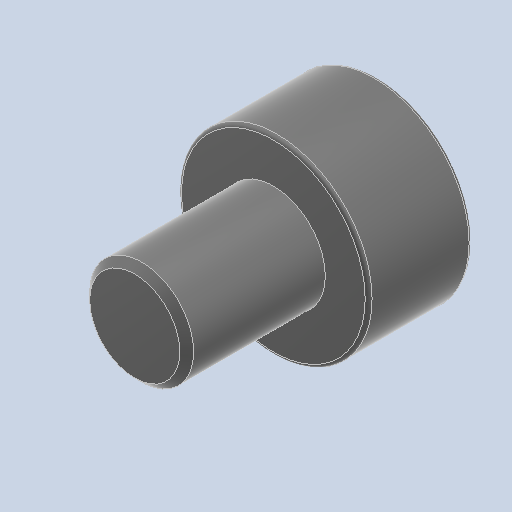
# Autodesk Inventor part: M3 x 4mm FHCS
Saved by Autodesk Inventor 2022 (Build 260153000, 153)
## iProperties
Created: 2021-10-06
Part Number: M3 x 4mm FHCS
Material: Stainless Steel
Document SubType Name: Modeling
Designer: Administrator
Density: 8 g/cm^3
Appearance: Smooth - Black
Mass: 0.890655 g
Surface Area: 1.98084 cm^2
Volume: 0.111332 cm^3
Title: DIN 912 M3 8 mm
Author: Administrator
Autodesk Inventor part; units mm, degrees
ref_plane "YZ Plane" through (0, 0, 0) normal (1, 0, 0) x (0, 1, 0)
ref_plane "XZ Plane" through (0, 0, 0) normal (0, 1, 0) x (-1, 0, 0)
ref_plane "Work Plane1" through (0, 0, -3) normal (0, 0, 1) x (1, 0, 0)
sketch "Sketch1" plane through (0, 0, -3) normal (0, 0, 1) x (1, 0, 0)
  circle A0 centre (0, 0) radius 2.75
  constraints: 1 centre point
extrude "Extrusion3" add sketch "Sketch1" along normal blind 3
fillet "Fillet1" radius 0.1 2 edges at (-2.75, 0, -3) (-2.75, 0, 0)
sketch "Sketch2" plane through (0, 0, -3) normal (0, 0, 1) x (1, 0, 0)
  line L0 (-0.7217, 1.25) -> (0.7217, 1.25)
  line L1 (0.7217, -1.25) -> (-0.7217, -1.25)
  line L2 (-0.7217, -1.25) -> (-1.4434, 0)
  line L3 (0.7217, 1.25) -> (1.4434, 0)
  line L4 (-1.4434, 0) -> (-0.7217, 1.25)
  line L5 (1.4434, 0) -> (0.7217, -1.25)
  constraints: 12 end point, 5 equal length, 2 horizontal
extrude "Extrusion2" cut sketch "Sketch2" along normal blind 3
sketch "Sketch3" plane through (0, 0, 0) normal (0, 0, 1) x (1, 0, 0)
  circle A0 centre (0, 0) radius 1.5
  constraints: 1 centre point
extrude "Extrusion1" add sketch "Sketch3" along normal blind 4
chamfer "Chamfer1" distance 0.2 angle 45 1 edges at (-1.5, 0, 4)
body "Solid3"
